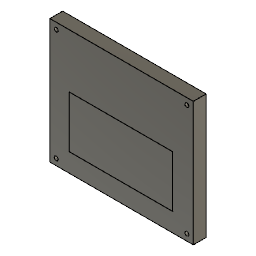
Assembled with pcb (Autodesk Fusion 360 archive; units mm, degrees)
design "Back-display"
part number: 2026-02-05-20-27-14-774
Autodesk Fusion 360 part; units mm, degrees
sketch "Sketch1" plane through (0, 0, 0) normal (0, 1, 0) x (1, 0, 0)
  line L0 (48.2925, -50) -> (-62.7075, -50)
  line L1 (-62.7075, -50) -> (-62.7075, 46.2)
  line L2 (-62.7075, 46.2) -> (48.2925, 46.2)
  line L3 (48.2925, 46.2) -> (48.2925, -50)
  circle A0 centre (43.2925, -45) radius 1.5
  circle A1 centre (-57.7075, -45) radius 1.5
  circle A2 centre (-57.7075, 41.2) radius 1.5
  circle A3 centre (43.2925, 41.2) radius 1.5
  line L4 (32.2706, -8.2971) -> (-47.7294, -8.2971)
  line L5 (-47.7294, -8.2971) -> (-47.7294, 31.7029)
  line L6 (-47.7294, 31.7029) -> (32.2706, 31.7029)
  line L7 (32.2706, 31.7029) -> (32.2706, -8.2971)
  dimension "d1" = 111
  dimension "d2" = 96.2
  dimension "d3" = 3
  dimension "d4" = 5
  dimension "d5" = 5
  dimension "d6" = 3
  dimension "d7" = 5
  dimension "d8" = 5
  dimension "d9" = 3
  dimension "d10" = 5
  dimension "d11" = 5
  dimension "d12" = 3
  dimension "d13" = 5
  dimension "d14" = 5
  dimension "d15" = 40
  dimension "d16" = 80
  constraint horizontal L0
  constraint vertical L1
  constraint horizontal L2
  constraint vertical L3
  constraint horizontal L4
  constraint vertical L5
  constraint horizontal L6
  constraint vertical L7
  measures "d1" distance of L1 L3
  measures "d2" distance of L0 L2
  measures "d3" diameter of A0
  measures "d4" distance of L3 A0.centre
  measures "d5" distance of L0 A0.centre
  measures "d6" diameter of A1
  measures "d7" distance of L1 A1.centre
  measures "d8" distance of L0 A1.centre
  measures "d9" diameter of A2
  measures "d10" distance of L1 A2.centre
  measures "d11" distance of L2 A2.centre
  measures "d12" diameter of A3
  measures "d13" distance of L2 A3.centre
  measures "d14" distance of L3 A3.centre
  measures "d15" distance of L4 L6
  measures "d16" distance of L5 L7
extrude "Extrude1" add sketch "Sketch1" along normal blind 10 makes body 1
extrude "Extrude2" add sketch "Sketch1" along normal blind 4 separate body contours L4 L5 L6 L7 makes body 2
